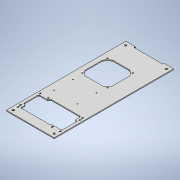
# Autodesk Inventor part: bottom_panel2
Saved by Autodesk Inventor 2022 (Build 260153000, 153)
## iProperties
Created: 2021-05-09
Part Number: bottom_panel2
Material: Generic
Document SubType Name: Modeling
Designer: gisen
Density: 1 g/cm^3
Appearance: Default
Author: gisen
Autodesk Inventor part; units mm, degrees
ref_plane "YZ Plane" through (0, 0, 0) normal (1, 0, 0) x (0, 1, 0)
ref_plane "XZ Plane" through (0, 0, 0) normal (0, 1, 0) x (-1, 0, 0)
ref_plane "XY Plane" through (0, 0, 0) normal (0, 0, 1) x (1, 0, 0)
sketch "Sketch1" plane through (0, 0, 0) normal (0, 0, 1) x (1, 0, 0)
  line L0 (-78, 195) -> (78, 195)
  line L1 (78, 195) -> (78, -195)
  line L2 (78, -195) -> (-78, -195)
  line L3 (-78, -195) -> (-78, 195)
  line L4 (-78, 195) -> (78, -195) construction
  line L5 (78, 195) -> (-78, -195) construction
  arc A0 (-64.4298, -185.2577) -> (-68.2577, -181.4298) centre (-66, -183) ccw
  arc A1 (-69.8472, -183.7153) -> (-66.7153, -186.8472) centre (-68, -185) ccw
  line L6 (-64.4298, -185.2577) -> (-66.7153, -186.8472)
  line L7 (-68.2577, -181.4298) -> (-69.8472, -183.7153)
  line L8 (0, 12.0891) -> (0, -12.7178)
  line L9 (-14.9134, -0.3143) -> (28.4633, -0.3143)
  arc A2 (68.2577, -181.4298) -> (64.4298, -185.2577) centre (66, -183) ccw
  arc A3 (66.7153, -186.8472) -> (69.8472, -183.7153) centre (68, -185) ccw
  line L10 (64.4298, -185.2577) -> (66.7153, -186.8472)
  line L11 (68.2577, -181.4298) -> (69.8472, -183.7153)
  arc A4 (-68.2577, 180.8012) -> (-64.4298, 184.629) centre (-66, 182.3713) ccw
  arc A5 (-66.7153, 186.2185) -> (-69.8472, 183.0866) centre (-68, 184.3713) ccw
  line L12 (-64.4298, 184.629) -> (-66.7153, 186.2185)
  line L13 (-68.2577, 180.8012) -> (-69.8472, 183.0866)
  arc A6 (64.4298, 184.629) -> (68.2577, 180.8012) centre (66, 182.3713) ccw
  line L14 (68.2577, 180.8012) -> (69.8472, 183.0866)
  line L15 (64.4298, 184.629) -> (66.7153, 186.2185)
  arc A7 (69.8472, 183.0866) -> (66.7153, 186.2185) centre (68, 184.3713) ccw
  point P0 (0, 0)
  dimension "d507" = 390
  dimension "d508" = 156
  dimension "d513" = 5.5
  dimension "d514" = 4.5
  dimension "d515" = 10
  dimension "d516" = 10
  dimension "d517" = 12
  dimension "d518" = 12
  constraints: 32 end point, 18 symmetric about line, 16 point on circle, 8 centre point, 4 tangent, 2 horizontal, 2 midpoint, 2 parallel, 1 perpendicular, 1 vertical, 6 other
  measures "d507" distance of L0.end L1.end
  measures "d508" distance of L1.end L2.end
  measures "d513" diameter of A0
  measures "d514" diameter of A1
  measures "d515" distance from line of L2 A1.centre
  measures "d516" distance from line of L3 A1.centre
  measures "d517" distance from line of L2 A0.centre
  measures "d518" distance from line of L3 A0.centre
extrude "Extrusion2" add sketch "Sketch1" along normal blind 3
sketch "Sketch3" plane through (0, 0, 3) normal (0, 0, 1) x (1, 0, 0)
  line L0 (-66, -98.4) -> (-40.5, -98.4)
  arc A0 (-71.75, -94.4) -> (-68.25, -94.4) centre (-70, -94.4) ccw
  arc A1 (-68.25, -91.4) -> (-71.75, -91.4) centre (-70, -91.4) ccw
  line L1 (-71.75, -94.4) -> (-71.75, -91.4)
  line L2 (-68.25, -91.4) -> (-68.25, -94.4)
  arc A2 (-66, -98.4) -> (-69, -101.4) centre (-66, -101.4) ccw
  line L3 (-69, -145.9) -> (-69, -101.4)
  line L4 (-45.75, -94.2) -> (-45.75, -91.2)
  arc A3 (-42.25, -91.2) -> (-45.75, -91.2) centre (-44, -91.2) ccw
  line L5 (-42.25, -91.2) -> (-42.25, -94.2)
  arc A4 (-45.75, -94.2) -> (-42.25, -94.2) centre (-44, -94.2) ccw
  arc A5 (-34.5, -91.6) -> (-37.5, -94.6) centre (-34.5, -94.6) ccw
  arc A6 (-40.5, -98.4) -> (-37.5, -95.4) centre (-40.5, -95.4) ccw
  line L6 (-37.5, -95.4) -> (-37.5, -94.6)
  line L7 (-34.5, -91.6) -> (58.5, -91.6)
  arc A7 (61.5, -94.6) -> (58.5, -91.6) centre (58.5, -94.6) ccw
  line L8 (66.25, -94.4) -> (66.25, -91.4)
  arc A8 (69.75, -91.4) -> (66.25, -91.4) centre (68, -91.4) ccw
  line L9 (69.75, -91.4) -> (69.75, -94.4)
  arc A9 (66.25, -94.4) -> (69.75, -94.4) centre (68, -94.4) ccw
  arc A10 (71.75, -101.2) -> (68.25, -101.2) centre (70, -101.2) ccw
  line L10 (68.25, -104.2) -> (68.25, -101.2)
  line L11 (71.75, -101.2) -> (71.75, -104.2)
  arc A11 (68.25, -104.2) -> (71.75, -104.2) centre (70, -104.2) ccw
  line L12 (61.5, -94.6) -> (61.5, -107.7)
  arc A12 (61.5, -107.7) -> (64.5, -110.7) centre (64.5, -107.7) ccw
  line L13 (64.5, -110.7) -> (66, -110.7)
  arc A13 (69, -113.7) -> (66, -110.7) centre (66, -113.7) ccw
  line L14 (69, -113.7) -> (69, -158.4)
  arc A14 (66, -161.4) -> (69, -158.4) centre (66, -158.4) ccw
  line L15 (66, -161.4) -> (39.9991, -161.4)
  arc A15 (71.75, -165.2) -> (68.25, -165.2) centre (70, -165.2) ccw
  line L16 (68.25, -168.2) -> (68.25, -165.2)
  line L17 (71.75, -165.2) -> (71.75, -168.2)
  arc A16 (68.25, -168.2) -> (71.75, -168.2) centre (70, -168.2) ccw
  arc A17 (39.9991, -161.4) -> (37.2495, -163.2) centre (39.9991, -164.4) ccw
  arc A18 (34.5, -165) -> (37.2495, -163.2) centre (34.5, -162) ccw
  line L18 (34.5, -165) -> (-58.5, -165)
  line L19 (42.25, -168.4) -> (42.25, -165.4)
  arc A19 (45.75, -165.4) -> (42.25, -165.4) centre (44, -165.4) ccw
  line L20 (45.75, -165.4) -> (45.75, -168.4)
  arc A20 (42.25, -168.4) -> (45.75, -168.4) centre (44, -168.4) ccw
  arc A21 (-61.5, -162) -> (-58.5, -165) centre (-58.5, -162) ccw
  line L21 (-61.5, -162) -> (-61.5, -151.9)
  arc A22 (-61.5, -151.9) -> (-64.5, -148.9) centre (-64.5, -151.9) ccw
  arc A23 (-69, -145.9) -> (-66, -148.9) centre (-66, -145.9) ccw
  line L22 (-64.5, -148.9) -> (-66, -148.9)
  arc A24 (-68, -155.4) -> (-72, -155.4) centre (-70, -155.4) ccw
  line L23 (-68, -155.4) -> (-68, -158.4)
  line L24 (-72, -158.4) -> (-72, -155.4)
  arc A25 (-72, -158.4) -> (-68, -158.4) centre (-70, -158.4) ccw
  arc A26 (-66.25, -165.2) -> (-69.75, -165.2) centre (-68, -165.2) ccw
  line L25 (-69.75, -168.2) -> (-69.75, -165.2)
  line L26 (-66.25, -165.2) -> (-66.25, -168.2)
  arc A27 (-69.75, -168.2) -> (-66.25, -168.2) centre (-68, -168.2) ccw
  line L27 (-78, -195) -> (78, -195) projected
  point P0 (0, 0)
  dimension "d524" = 1.75
  dimension "d525" = 3
  dimension "d526" = 2
  dimension "d527" = 2
  dimension "d528" = 2.75
  dimension "d529" = 10.25
  dimension "d530" = 26
  dimension "d531" = 109.25
  dimension "d532" = 114
  dimension "d533" = 133.25
  dimension "d534" = 138
  dimension "d535" = 139.75
  dimension "d536" = 140
  dimension "d537" = 140.75
  dimension "d538" = 50.7
  dimension "d539" = 19.1
  dimension "d540" = 54.3
  dimension "d541" = 12.3
  dimension "d542" = 38.2
  dimension "d543" = 9.5
  dimension "d544" = 6.5
  dimension "d545" = 54.5
  dimension "d546" = 57.5
  dimension "d547" = 19.3
  dimension "d548" = 16.3
  dimension "d549" = 54.7
  dimension "d550" = 57.7
  dimension "d551" = 31.7509
  dimension "d552" = 19.5
  dimension "d553" = 16.5
  dimension "d554" = 54.5
  dimension "d555" = 44.7
  dimension "d556" = 137.75
  dimension "d557" = 57.5
  dimension "d558" = 16.3
  dimension "d559" = 139
  dimension "d560" = 19.3
  dimension "d561" = 139
  dimension "d562" = 47.7
  dimension "d563" = 30
  constraints: 56 point on circle, 54 end point, 46 tangent, 28 centre point, 25 equal radius, 19 parallel, 6 perpendicular
  measures "d524" radius of A10
  measures "d525" radius of A13
  measures "d526" radius of A24
  measures "d527" distance between parallel lines of L9 L11
  measures "d528" distance between parallel lines of L14 L11
  measures "d529" distance between parallel lines of L12 L11
  measures "d530" distance between parallel lines of L11 L20
  measures "d531" distance between parallel lines of L6 L11
  measures "d532" distance between parallel lines of L11 L5
  measures "d533" distance between parallel lines of L21 L11
  measures "d534" distance between parallel lines of L26 L11
  measures "d535" distance between parallel lines of L23 L11
  measures "d536" distance between parallel lines of L11 L2
  measures "d537" distance between parallel lines of L3 L11
  measures "d538" distance between parallel lines of L13 L15
  measures "d539" distance between parallel lines of L7 L13
  measures "d540" distance between parallel lines of L18 L13
  measures "d541" distance between parallel lines of L13 L0
  measures "d542" distance between parallel lines of L22 L13
  measures "d543" distance from line of L11.start L13
  measures "d544" distance from line of L11.end L13
  measures "d545" distance from line of L17.start L13
  measures "d546" distance from line of L17.end L13
  measures "d547" distance from line of L9.start L13
  measures "d548" distance from line of L9.end L13
  measures "d549" distance from line of L20.start L13
  measures "d550" distance from line of L20.end L13
  measures "d551" distance from line of L15.end L11
  measures "d552" distance from line of L5.start L13
  measures "d553" distance from line of L5.end L13
  measures "d554" distance from line of L26.start L13
  measures "d555" distance from line of L23.start L13
  measures "d556" distance from line of A27.centre L9
  measures "d557" distance from line of A27.centre L13
  measures "d558" distance from line of L2.end L13
  measures "d559" distance from line of A1.centre L14
  measures "d560" distance from line of A1.centre L13
  measures "d561" distance from line of A25.centre L14
  measures "d562" distance from line of A25.centre L13
  measures "d563" distance between parallel lines of L27 L18
extrude "Extrusion3" cut sketch "Sketch3" against normal through all
sketch "Sketch5" plane through (0, 0, 3) normal (0, 0, 1) x (1, 0, 0)
  line L0 (78, -195) -> (78, 195) projected
  line L1 (78, 195) -> (-78, 195) projected
  line L2 (-45.9537, 120.0288) -> (9.9537, 120.0288)
  line L3 (26.7, 103.4765) -> (26.7, 46.5235)
  line L4 (10.9861, 30.6288) -> (-46.9861, 30.6288)
  line L5 (-62.7, 46.5235) -> (-62.7, 103.4765)
  line L6 (-62.3588, 119.7124) -> (26.6856, 29.9582) construction
  line L7 (26.7, 119.7) -> (-62.7, 30.3) construction
  arc A0 (-45.9537, 120.0288) -> (-62.7, 103.4765) centre (-18, 75) ccw
  arc A1 (26.7, 103.4765) -> (9.9537, 120.0288) centre (-18, 75) ccw
  arc A2 (-62.7, 46.5235) -> (-46.9861, 30.6288) centre (-18, 75) ccw
  arc A3 (10.9861, 30.6288) -> (26.7, 46.5235) centre (-18, 75) ccw
  circle A4 centre (-59.25, 116.5788) radius 2.25
  circle A5 centre (-59.25, 34.0788) radius 2.25
  circle A6 centre (23.25, 116.5788) radius 2.25
  circle A7 centre (23.25, 34.0788) radius 2.25
  point P0 (0, 0)
  dimension "d566" = 96
  dimension "d568" = 120
  dimension "d571" = 89.4
  dimension "d572" = 89.4
  dimension "d573" = 3.45
  dimension "d574" = 3.45
  dimension "d575" = 4.5
  dimension "d578" = 82.5
  dimension "d581" = 82.5
  constraints: 12 end point, 8 centre point, 8 point on circle, 2 horizontal, 2 parallel, 2 point on line, 1 coincident, 1 midpoint, 1 perpendicular, 1 vertical, 6 other
  measures "d566" distance from line of L0 point (-18, 75)
  measures "d568" distance from line of L1 point (-18, 75)
  measures "d571" distance between parallel lines of L4 L2
  measures "d572" distance between parallel lines of L3 L5
  measures "d573" distance from line of L2 A4.centre
  measures "d574" distance from line of A4.centre L5
  measures "d575" diameter of A4
  measures "d578" distance of A4.centre A5.centre
  measures "d581" distance of A4.centre A6.centre
extrude "Extrusion4" cut sketch "Sketch5" against normal up to surface (3 mm away)
sketch "Sketch7" plane through (0, 0, 3) normal (0, 0, 1) x (1, 0, 0)
  line L0 (78, 195) -> (-78, 195) projected
  line L1 (-46.75, 195) -> (46.75, 195)
  line L2 (46.75, 195) -> (46.75, 190.5)
  line L3 (46.75, 190.5) -> (-46.75, 190.5)
  line L4 (-46.75, 190.5) -> (-46.75, 195)
  line L5 (78, -195) -> (78, 195) projected
  point P0 (0, 0)
  dimension "d586" = 93.5
  dimension "d587" = 4.5
  dimension "d588" = 156
  dimension "d589" = 31.25
  constraints: 8 end point, 2 parallel, 1 horizontal, 1 perpendicular, 1 point on line
  measures "d586" distance between parallel lines of L2 L4
  measures "d587" distance between parallel lines of L0 L3
  measures "d588" distance of L0.start L0.end
  measures "d589" distance between parallel lines of L5 L2
extrude "Extrusion5" cut sketch "Sketch7" against normal up to surface (3 mm away)
sketch "Sketch8" plane through (0, 0, 3) normal (0, 0, 1) x (1, 0, 0)
  arc A0 (-62.7, 46.5235) -> (-46.9861, 30.6288) centre (-18, 75) ccw projected
  line L0 (-78, 195) -> (-78, -195) projected
  line L1 (-78, -195) -> (78, -195) projected
  line L2 (10.9861, 30.6288) -> (-46.9861, 30.6288) projected
  point P0 (0, 0)
  point P1 (-56.3, -61.0912)
  point P2 (-56.3, 0.6288)
  point P3 (20.3, -61.0912)
  point P4 (20.3, 0.6288)
  dimension "d592" = 60
  dimension "d598" = 61.72
  dimension "d601" = 76.6
  dimension "d604" = 21.7
  dimension "d605" = 30
  constraints: 1 horizontal, 1 vertical, 3 other
  measures "d592" distance from line of A0.centre L0
  measures "d598" distance of point (-56.3, -61.091) point (-56.3, 0.629)
  measures "d601" distance of point (-56.3, -61.091) point (20.3, -61.091)
  measures "d604" distance from line of point (-56.3, -61.091) L0
  measures "d605" distance from line of point (-56.3, 0.629) L2
hole "Hole2" at (-56.3, -61.0912, 3) at (-56.3, 0.6288, 3) at (20.3, -61.0912, 3) at (20.3, 0.6288, 3) direction (0, 0, -1) diameter 3.2 end through all
sketch "Sketch9" plane through (0, 0, 3) normal (0, 0, 1) x (1, 0, 0)
  line L0 (-46.75, 195) -> (-78, 195) projected
  line L1 (-46.75, 190.5) -> (-46.75, 195) projected
  line L2 (46.75, 190.5) -> (-46.75, 190.5) projected
  line L3 (46.75, 195) -> (46.75, 190.5) projected
  line L4 (78, 195) -> (46.75, 195) projected
  circle A0 centre (-45.6363, 191.6137) radius 1.575
  circle A1 centre (45.6363, 191.6137) radius 1.575
  point P0 (0, 0)
  point P1 (-44.5226, 190.5)
  point P2 (-46.75, 192.7274)
  point P3 (44.5226, 190.5)
  point P4 (46.75, 192.7274)
  point P5 (-46.75, 192.7274)
  dimension "d620" = 3.15
  dimension "d622" = 2.2274
  dimension "d624" = 2.2274
  dimension "d625" = 3.15
  dimension "d626" = 2.2274
  constraints: 5 point on circle, 2 centre point, 2 coincident, 2 point on line
  measures "d620" diameter of A0
  measures "d622" distance of A0.end point (-46.75, 190.5)
  measures "d624" distance of point (-46.75, 190.5) point (-46.75, 192.727)
  measures "d625" diameter of A1
  measures "d626" distance of A1.start A1.end
extrude "Extrusion6" cut sketch "Sketch9" against normal up to surface (3 mm away) contours A0 L1 | L2 A0 | A1 L2 | L3 A1
body "Solid2"
